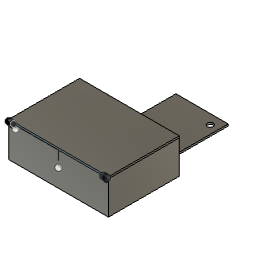
cc_sfs_adapter (Autodesk Fusion 360 design; units mm, degrees)
Autodesk Fusion 360 part; units mm, degrees
note: some values were not read from the file. Chosen so that the rebuilt part matches the saved one: which bodies a step acts on.
sketch "Sketch1" plane through (0, 0, 0) normal (0, 0, 1) x (1, 0, 0)
  line L0 (0, 0) -> (35, 0) construction
  line L1 (35, 0) -> (35, 40.5) construction
  line L2 (35, 40.5) -> (0, 40.5) construction
  line L3 (0, 40.5) -> (0, 0) construction
  line L4 (0, 0) -> (6, 0) construction
  line L5 (6, 0) -> (6, 5.5) construction
  line L6 (6, 5.5) -> (0, 5.5) construction
  line L7 (0, 5.5) -> (0, 0) construction
  line L8 (35, 40.5) -> (29.5, 40.5) construction
  line L9 (29.5, 40.5) -> (29.5, 34) construction
  line L10 (29.5, 34) -> (35, 34) construction
  line L11 (35, 34) -> (35, 40.5) construction
  circle A0 centre (29.5, 34) radius 2
  circle A1 centre (6, 5.5) radius 1.875
  line L12 (0, 40.5) -> (11.5, 40.5) construction
  line L13 (11.5, 40.5) -> (11.5, 0) construction
  line L14 (11.5, 0) -> (11.5, -5) construction
  line L15 (11.5, -5) -> (36.5, -5) construction
  line L16 (36.5, -5) -> (36.5, 48) construction
  line L17 (36.5, 48) -> (11.5, 48) construction
  line L18 (11.5, 48) -> (11.5, -5) construction
  line L19 (36.5, -5) -> (46.5, -5) construction
  line L20 (46.5, -5) -> (-17.5, -5)
  line L21 (-17.5, -5) -> (-17.5, -50)
  line L22 (-17.5, -50) -> (46.5, -50)
  line L23 (46.5, -50) -> (46.5, -5)
  line L24 (0, 40.5) -> (0, -5)
  line L25 (0, 40.5) -> (35, 40.5)
  line L26 (35, 40.5) -> (35, -5)
  dimension "d1" = 35
  dimension "d2" = 40.5
  dimension "d3" = 6
  dimension "d4" = 5.5
  dimension "d5" = 5.5
  dimension "d6" = 6.5
  dimension "d7" = 4
  dimension "d8" = 3.75
  dimension "d9" = 11.5
  dimension "d10" = 5
  dimension "d11" = 25
  dimension "d12" = 53
  dimension "d13" = 10
  dimension "d14" = 64
  dimension "d15" = 45
  constraint horizontal L0
  constraint vertical L1
  constraint horizontal L2
  constraint vertical L3
  constraint coincident L0.start L3.end
  constraint horizontal L4
  constraint vertical L5
  constraint horizontal L6
  constraint vertical L7
  constraint horizontal L8
  constraint vertical L9
  constraint horizontal L10
  constraint vertical L11
  constraint coincident L9.end L10.start
  constraint coincident L5.end L6.start
  constraint perpendicular L3 L12
  constraint coincident L0 L13.end
  constraint perpendicular L0 L13
  constraint perpendicular L0 L14
  constraint horizontal L15
  constraint vertical L16
  constraint horizontal L17
  constraint vertical L18
  constraint perpendicular L16 L19
  constraint horizontal L20
  constraint vertical L21
  constraint horizontal L22
  constraint vertical L23
  constraint coincident L20 L24.end
  constraint perpendicular L20 L24
  constraint coincident L20 L26.end
  measures "d1" distance of L0.start L0.end
  measures "d2" distance of L0.start L2.end
  measures "d3" distance of L0.start L4.end
  measures "d4" distance of L0.start L6.end
  measures "d5" distance of L1.end L8.end
  measures "d6" distance of L1.end L10.end
  measures "d7" diameter of A0
  measures "d8" diameter of A1
  measures "d9" distance of L2.end L12.end
  measures "d10" distance of L13.end L14.end
  measures "d11" distance of L14.end L15.end
  measures "d12" distance of L14.end L17.end
  measures "d13" distance of L15.end L19.end
  measures "d14" distance of L19.end L20.end
  measures "d15" distance of L19.end L22.end
extrude "Extrude1" add sketch "Sketch1" along normal blind 1.2 makes body 1
sketch "Sketch2" plane through (0, 0, 1.2) normal (0, 0, 1) x (-1, 0, 0)
  circle A0 centre (-6, -5.5) radius 1.875
  circle A1 centre (-29.5, -34) radius 2
  line L0 (0, -40.5) -> (0, 5)
  line L1 (0, 5) -> (17.5, 5)
  line L2 (17.5, 5) -> (17.5, 50)
  line L3 (17.5, 50) -> (-46.5, 50)
  line L4 (-46.5, 50) -> (-46.5, 5)
  line L5 (-46.5, 5) -> (-35, 5)
  line L6 (-35, 5) -> (-35, -40.5)
  line L7 (-35, -40.5) -> (0, -40.5)
  circle A2 centre (-6, -5.5) radius 4.875
  line L8 (17.5, 5) -> (-46.5, 5)
  line L9 (-46.5, 5) -> (-46.5, 50)
  line L10 (-46.5, 50) -> (17.5, 50)
  line L11 (17.5, 50) -> (17.5, 5)
  dimension "d18" = 3
  constraint horizontal L8
  constraint vertical L9
  constraint horizontal L10
  constraint vertical L11
  constraint coincident L3.end L4.start
  constraint coincident L1.end L2.start
extrude "Extrude2" add sketch "Sketch2" along normal blind 5.6 contours A2 bodies 1
extrude "Extrude3" add 1 faces at (3.8333, -50, 0.4) along direction (0, -1, 0) blind 2.4 on bodies 1 bodies 1
extrude "Extrude4" add 1 faces at (46.5, -36.6, 0.8) along direction (1, 0, 0) blind 1.2 on bodies 1 bodies 1
extrude "Extrude5" add 1 faces at (-17.5, -36.6, 0.8) along direction (-1, 0, 0) blind 1.5 on bodies 1 bodies 1
sketch "Sketch3" plane through (0, 0, 1.2) normal (0, 0, 1) x (-1, 0, 0)
  circle A0 centre (-6, -5.5) radius 4.875
  circle A1 centre (-29.5, -34) radius 2
  line L0 (0, -40.5) -> (0, 5)
  line L1 (0, 5) -> (19, 5)
  line L2 (19, 5) -> (19, 52.4)
  line L3 (19, 52.4) -> (-47.7, 52.4)
  line L4 (-47.7, 52.4) -> (-47.7, 5)
  line L5 (-47.7, 5) -> (-35, 5)
  line L6 (-35, 5) -> (-35, -40.5)
  line L7 (-35, -40.5) -> (0, -40.5)
  line L8 (0, 5) -> (-35, 5)
  line L9 (0, 6.2) -> (-35, 6.2)
  line L10 (-46.5, 6.2) -> (-35, 6.2)
  line L11 (-46.5, 51.2) -> (-46.5, 6.2)
  line L12 (17.8, 51.2) -> (-46.5, 51.2)
  line L13 (17.8, 6.2) -> (17.8, 51.2)
  line L14 (0, 6.2) -> (17.8, 6.2)
  line L15 (-46.5, 51.2) -> (-46.5, 48.2) construction
  line L16 (-46.5, 48.2) -> (-41.5, 48.2) construction
  line L17 (-41.5, 48.2) -> (-31, 48.2)
  line L18 (-31, 48.2) -> (-31, 41.7)
  line L19 (-31, 41.7) -> (-41.5, 41.7)
  line L20 (-41.5, 41.7) -> (-41.5, 48.2)
  line L21 (-46.5, 51.2) -> (-46.5, 48.5) construction
  line L22 (-46.5, 48.5) -> (-43.5, 48.5) construction
  circle A2 centre (-43.5, 48.5) radius 0.95
  line L23 (-46.5, 6.2) -> (-43.5, 6.2) construction
  line L24 (-43.5, 6.2) -> (-43.5, 8.9) construction
  line L25 (-43.5, 8.9) -> (-46.5, 8.9) construction
  line L26 (-46.5, 8.9) -> (-46.5, 6.2) construction
  circle A3 centre (-43.5, 8.9) radius 0.95
  line L27 (-43.5, 8.9) -> (1, 8.9) construction
  line L28 (-43.5, 48.5) -> (1, 48.5) construction
  circle A4 centre (1, 8.9) radius 0.95
  circle A5 centre (1, 48.5) radius 0.95
  dimension "d27" = -1.2
  dimension "d28" = 3
  dimension "d29" = 5
  dimension "d30" = 10.5
  dimension "d31" = 6.5
  dimension "d32" = 2.7
  dimension "d33" = 3
  dimension "d34" = 1.9
  dimension "d35" = 3
  dimension "d36" = 2.7
  dimension "d37" = 1.9
  dimension "d38" = 44.5
  dimension "d39" = 44.5
  dimension "d40" = 1.9
  dimension "d41" = 1.9
  constraint coincident L0.end L1.start
  constraint coincident L5.end L6.start
  constraint perpendicular L12 L15
  constraint perpendicular L11 L16
  constraint horizontal L17
  constraint vertical L18
  constraint horizontal L19
  constraint vertical L20
  constraint perpendicular L12 L21
  constraint perpendicular L21 L22
  constraint coincident L22.end A2.centre
  constraint horizontal L23
  constraint vertical L24
  constraint horizontal L25
  constraint vertical L26
  constraint coincident L24.end L25.start
  constraint perpendicular L24 L27
  constraint parallel L22 L28
  constraint coincident L27.end A4.centre
  constraint coincident L28.end A5.centre
  measures "d28" distance of L11.start L15.end
  measures "d29" distance of L15.end L16.end
  measures "d30" distance of L16.end L17.end
  measures "d31" distance of L16.end L19.end
  measures "d32" distance of L11.start L21.end
  measures "d33" distance of L21.end L22.end
  measures "d34" diameter of A2
  measures "d35" distance of L10.start L23.end
  measures "d36" distance of L10.start L25.end
  measures "d37" diameter of A3
  measures "d38" distance of L24.end L27.end
  measures "d39" distance of L22.end L28.end
  measures "d40" diameter of A4
  measures "d41" diameter of A5
extrude "Extrude6" cut sketch "Sketch3" against normal blind 1.2 contours L17 L18 L19 L20 bodies 1
extrude "Extrude7" add sketch "Sketch3" along normal blind 21 contours L1 L2 L3 L4 L5 L8 bodies 1
extrude "Extrude8" add sketch "Sketch3" along normal blind 7.5 draft -2 contours A2 | A3 | A4 | A5 bodies 1
sketch "Sketch4" plane through (0, -6.2, 0) normal (0, -1, 0) x (1, 0, 0)
  line L0 (35, 1.2) -> (46.5, 1.2)
  line L1 (46.5, 1.2) -> (46.5, 22.2)
  line L2 (46.5, 22.2) -> (35, 22.2)
  line L3 (35, 22.2) -> (35, 1.2)
  line L4 (46.5, 22.2) -> (30.5, 22.2)
  line L5 (30.5, 22.2) -> (20.5, 22.2)
  line L6 (20.5, 22.2) -> (20.5, 13.2)
  line L7 (20.5, 13.2) -> (30.5, 13.2)
  line L8 (30.5, 13.2) -> (30.5, 22.2)
  dimension "d48" = 16
  dimension "d49" = 9
  dimension "d50" = 10
  constraint coincident L1.end L2.start
  constraint perpendicular L1 L4
  constraint horizontal L5
  constraint vertical L6
  constraint horizontal L7
  constraint vertical L8
  measures "d48" distance of L1.end L4.end
  measures "d49" distance of L4.end L7.end
  measures "d50" distance of L6.end L7.end
extrude "Extrude9" cut sketch "Sketch4" against normal blind 1.2 contours L5 L6 L7 L8 bodies 1
extrude "Extrude10" add sketch "Sketch3" along normal blind 1.2 from surface at 21 separate body contours L1 L2 L3 L4 L5 L8 | L9 L10 L11 L12 L13 L14 | L17 L18 L19 L20 | A2 | A3 | A4 | A5 makes body 2
sketch "Sketch5" plane through (0, -52.4, 0) normal (0, -1, 0) x (1, 0, 0)
  line L0 (-19, 22.2) -> (47.7, 22.2)
  line L1 (47.7, 22.2) -> (47.7, 23.4)
  line L2 (47.7, 23.4) -> (-19, 23.4)
  line L3 (-19, 23.4) -> (-19, 22.2)
  line L4 (-19, 22.2) -> (-17.7, 22.2) construction
  line L5 (-17.7, 22.2) -> (-17.7, 21.2)
  line L6 (-17.7, 21.2) -> (-17.7, 20.6) construction
  line L7 (-17.7, 20.6) -> (-17.7, 20) construction
  line L8 (-17.7, 20.6) -> (-18.3, 20.6) construction
  line L9 (-18.3, 20.6) -> (-17.7, 21.2)
  line L10 (-18.3, 20.6) -> (-17.7, 20)
  line L11 (-17.7, 20) -> (-16.7, 20)
  line L12 (-16.7, 20) -> (-15.8993, 22.2)
  line L13 (-16.7, 20) -> (-14.3588, 20) construction
  line L14 (-19, 22.2) -> (14.35, 22.2) construction
  line L15 (14.35, 22.2) -> (14.35, 12) construction
  line L16 (-17.85, 22.2) -> (-17.85, 21.2621)
  line L17 (-18.5121, 20.6) -> (-17.85, 21.2621)
  line L18 (-18.5121, 20.6) -> (-17.7621, 19.85)
  line L19 (-17.7621, 19.85) -> (-16.595, 19.85)
  line L20 (-16.595, 19.85) -> (-15.7583, 22.1487)
  line L21 (-15.7583, 22.1487) -> (-15.74, 22.2)
  line L22 (46.4, 22.2) -> (46.4, 21.2)
  line L23 (46.55, 22.2) -> (46.55, 21.2621)
  line L24 (47.2121, 20.6) -> (46.55, 21.2621)
  line L25 (47, 20.6) -> (46.4, 21.2)
  line L26 (47.2121, 20.6) -> (46.4621, 19.85)
  line L27 (47, 20.6) -> (46.4, 20)
  line L28 (46.4621, 19.85) -> (45.295, 19.85)
  line L29 (46.4, 20) -> (45.4, 20)
  line L30 (45.295, 19.85) -> (44.4583, 22.1487)
  line L31 (45.4, 20) -> (44.5993, 22.2)
  line L32 (44.4583, 22.1487) -> (44.44, 22.2)
  dimension "d56" = 1.3
  dimension "d57" = 1
  dimension "d58" = 0.6
  dimension "d59" = 0.6
  dimension "d60" = 0.6
  dimension "d61" = 1
  dimension "d62" = 70
  dimension "d63" = 0.15
  constraint coincident L0.start L3.end
  constraint perpendicular L3 L4
  constraint perpendicular L2 L5
  constraint perpendicular L0 L6
  constraint perpendicular L0 L7
  constraint perpendicular L7 L8
  constraint perpendicular L7 L11
  constraint horizontal L13
  constraint coincident L0 L12.end
  constraint midpoint L0 L14.end
  constraint perpendicular L14 L15
  constraint coincident L0 L21.end
  constraint symmetric L4.end L15 L22.start
  constraint symmetric L5.end L15 L22.end
  constraint symmetric L7.end L15 L27.end
  constraint symmetric L8.end L15 L25.start
  constraint symmetric L11.end L15 L29.end
  constraint symmetric L12.end L15 L31.end
  constraint symmetric L15 L16.start L23.start
  constraint symmetric L15 L16.end L23.end
  constraint symmetric L15 L17.start L24.start
  constraint symmetric L15 L18.end L26.end
  constraint symmetric L15 L19.end L28.end
  constraint symmetric L15 L20.end L30.end
  constraint symmetric L15 L21.end L32.end
  measures "d56" distance of L0.start L4.end
  measures "d57" distance of L4.end L5.end
  measures "d58" distance of L5.end L6.end
  measures "d59" distance of L6.end L7.end
  measures "d60" distance of L6.end L8.end
  measures "d61" distance of L7.end L11.end
  measures "d62" angle of L12 L13
sketch "Sketch6" plane through (0, 0, 22.2) normal (0, 0, -1) x (1, 0, 0)
  line L0 (-19, 52.4) -> (-19, 5)
  line L1 (-19, 5) -> (0, 5)
  line L2 (0, 5) -> (35, 5)
  line L3 (35, 5) -> (47.7, 5)
  line L4 (47.7, 5) -> (47.7, 52.4)
  line L5 (47.7, 52.4) -> (-19, 52.4)
  line L6 (-19, 28.7) -> (-18, 28.7)
  line L7 (-18, 28.7) -> (47.7, 28.7) construction
  constraint midpoint L0 L6.start
  constraint perpendicular L0 L6
  constraint midpoint L4 L7.end
extrude "Extrude11" add sketch "Sketch5" along normal blind 6 from surface at -10 separate body contours L0 L5 L9 L10 L11 L12 | L0 L22 L25 L27 L29 L31 makes body 3 at (-16.4331, -44.4, 20.7333) makes body 4 at (45.1331, -44.4, 20.7333)
ref_plane "WorkPlane1" through (14.35, -28.7, 22.8) normal (0, -1, 0) x (1, 0, 0)
mirror "Mirror1" about plane through (14.35, -28.7, 22.8) normal (0, -1, 0) of bodies 3 4 makes body 5 at (-16.4331, -13, 20.7333) makes body 6 at (45.1331, -13, 20.7333)
combine "Combine1" operation add target body 6 tool bodies 5 3 4 2
extrude "Extrude12" add sketch "Sketch5" along normal blind 6.3 from surface at -10.15 separate body contours L0 L5 L9 L10 L11 L12 L16 L17 L18 L19 L20 L21 | L0 L5 L9 L10 L11 L12 | L0 L22 L23 L24 L25 L26 L27 L28 L29 L30 L31 L32 | L0 L22 L25 L27 L29 L31 makes body 7 at (45.0161, -44.35, 20.6162) makes body 8 at (-16.3161, -44.35, 20.6162)
mirror "Mirror2" about plane through (14.35, -28.7, 22.8) normal (0, -1, 0) of bodies 8 7 makes body 9 at (45.0161, -10.95, 20.6162) makes body 10 at (-16.3161, -13.05, 20.6162)
combine "Combine2" operation cut target body 1 tool bodies 7 8 9 10
equation "d49 = 21 mm - 12 mm"
named bodies: "case", "lid"
